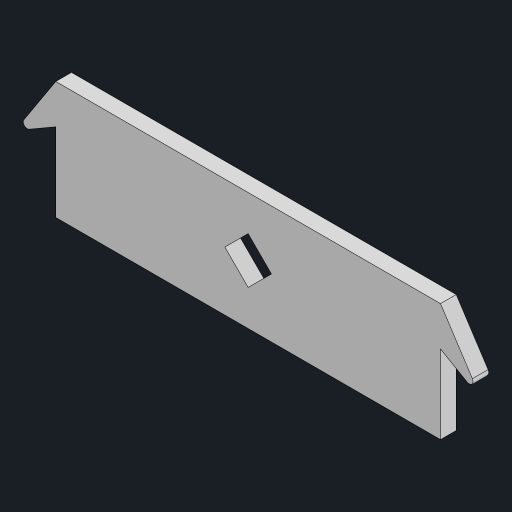
# Autodesk Inventor part: om_BackHolder_R
Saved by Autodesk Inventor 2023 (Build 270158000, 158)
## iProperties
Created: 2022-07-08
Part Number: om_BackHolder_R
Material: 一般
Document SubType Name: Modeling
Designer: legot
Density: 1 g/cm^3
Appearance: 既定
Author: legot
Autodesk Inventor part; units mm, degrees
ref_plane "YZ Plane" through (0, 0, 0) normal (1, 0, 0) x (0, 1, 0)
ref_plane "XZ Plane" through (0, 0, 0) normal (0, 1, 0) x (-1, 0, 0)
ref_plane "XY Plane" through (0, 0, 0) normal (0, 0, 1) x (1, 0, 0)
sketch "スケッチ1" plane through (0, 0, 0) normal (0, 0, 1) x (1, 0, 0)
  line L0 (-24.5, 7.5) -> (24.5, 7.5)
  line L1 (24.5, 7.5) -> (24.5, -7.5)
  line L2 (24.5, -7.5) -> (-24.5, -7.5)
  line L3 (-24.5, -7.5) -> (-24.5, 7.5)
  line L4 (-2.9698, 0) -> (0, 2.9698)
  line L5 (0, 2.9698) -> (2.9698, 0)
  line L6 (2.9698, 0) -> (0, -2.9698)
  line L7 (0, -2.9698) -> (-2.9698, 0)
  line L8 (-24.5, 7.5) -> (-28.5615, 1.2469)
  line L9 (-27.8922, 0.5415) -> (-24.5, 2.5)
  arc A0 (-28.5615, 1.2469) -> (-27.8922, 0.5415) centre (-28.1422, 0.9745) ccw
  line L10 (0, 7.5) -> (0, -7.5)
  point P0 (0, 0)
  point P1 (0, 0)
  point P2 (-24.5, 0)
  point P3 (-29.6962, -0.5)
  dimension "d0" = 4.2
  dimension "d1" = 15
  dimension "d2" = 49
  dimension "d3" = 6
  dimension "d4" = 60
  dimension "d5" = 5
  dimension "d6" = 0.5
  constraints: 22 end point, 4 parallel, 3 midpoint, 3 perpendicular, 3 point on line, 3 vertical alignment, 2 horizontal alignment, 2 point on circle, 2 tangent, 1 centre point, 1 coincident, 1 horizontal, 1 vertical
  measures "d0" distance of L4.start L4.end
  measures "d1" distance of L2.end L0.start
  measures "d2" distance of L0.start L0.end
  measures "d3" distance of point (-29.696, -0.5) L9.end
  measures "d4" angle of L3 L9
  measures "d5" distance of L0.start L9.end
  measures "d6" radius of A0
extrude "押し出し1" add sketch "スケッチ1" along normal blind 2 contours L0 L10 L4 L7 L2 L3 | L3 L9 A0 L8
mirror "ミラー1" about plane through (0, 2.9698, 0) normal (1, 0, 0) of "押し出し1"
